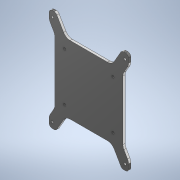
# Autodesk Inventor part: GPS - mount v2
Saved by Autodesk Inventor 2020.2 (Build 242310000, 310)
## iProperties
Created: 2020-08-26
Part Number: GPS - mount v2
Material: Generic
Document SubType Name: Modeling
Designer: Krishna Makhija
Density: 1 g/cm^3
Appearance: Default
Author: Krishna Makhija
Autodesk Inventor part; units mm, degrees
ref_plane "YZ Plane" through (0, 0, 0) normal (1, 0, 0) x (0, 1, 0)
ref_plane "XZ Plane" through (0, 0, 0) normal (0, 1, 0) x (-1, 0, 0)
ref_plane "XY Plane" through (0, 0, 0) normal (0, 0, 1) x (1, 0, 0)
sketch "Sketch3" plane through (0, 0, 0) normal (0, 0, 1) x (1, 0, 0)
  line L0 (52.5001, -67.5) -> (-52.5001, -67.5)
  line L1 (-52.5001, -67.5) -> (-52.5001, 67.5)
  line L2 (-52.5001, 67.5) -> (52.5001, 67.5)
  line L3 (52.5001, 67.5) -> (52.5001, -67.5)
  circle A0 centre (32, 32) radius 1.5
  circle A1 centre (-32, 32) radius 1.5
  circle A2 centre (-32, -32) radius 1.5
  circle A3 centre (32, -32) radius 1.5
  line L4 (30.5, 0) -> (-30.5, 0)
  line L5 (30.5, 45) -> (-30.5, 45)
  line L6 (30.5, 45) -> (43.4898, 67.5)
  line L7 (-30.5, 45) -> (-43.4888, 67.5)
  line L8 (30.5, -45) -> (-30.5, -45)
  line L9 (30.5, -45) -> (43.4898, -67.5)
  line L10 (-30.5, -45) -> (-43.4888, -67.5)
  line L11 (0, 42.0002) -> (0, -42)
  line L12 (45, 42.0002) -> (45, -42)
  line L13 (45, 42.0002) -> (52.5001, 54.9914)
  line L14 (45, -42) -> (52.5001, -54.9922)
  line L15 (-45, 42.0002) -> (-45, -42)
  line L16 (-45, 42.0002) -> (-52.5001, 54.9914)
  line L17 (-45, -42) -> (-52.5001, -54.9922)
  circle A4 centre (48, 60.0001) radius 1.428
  circle A5 centre (-48, 60.0001) radius 1.428
  circle A6 centre (48, -59.9999) radius 1.428
  circle A7 centre (-48, -59.9999) radius 1.428
  constraints: 36 end point, 8 centre point, 8 symmetric about line, 4 point on line, 3 horizontal, 2 parallel, 2 perpendicular
extrude "Extrusion2" add sketch "Sketch3" along normal blind 3 contours L0 L9 L8 L10 L1 L17 L15 L16 L2 L7 L5 L6 L3 L13 L12 L14 | L0 L10 L8 L9 | L14 L12 L13 L3 | L1 L16 L15 L17 | L6 L5 L7 L2 | A4 | A5 | A6 | A7
fillet "Fillet2" radius 4 4 edges at (-52.5001, 67.5, 1.5) (52.5001, 67.5, 1.5) (52.5001, -67.5, 1.5) (-52.5001, -67.5, 1.5)
extrude "Extrusion3" cut sketch "Sketch3" along normal blind 10 contours L0 L10 L8 L9 | L14 L12 L13 L3 | L1 L16 L15 L17 | L6 L5 L7 L2
fillet "Fillet3" radius 10 8 edges at (30.5, 45, 1.5) (-30.5, 45, 1.5) (30.5, -45, 1.5) (-30.5, -45, 1.5) (-52.5001, 54.9914, 1.5) (52.5001, -54.9922, 1.5) (-52.5001, -54.9922, 1.5) (52.5001, 54.9914, 1.5)
fillet "Fillet4" radius 10 4 edges at (45, 42.0002, 1.5) (45, -42, 1.5) (-45, -42, 1.5) (-45, 42.0002, 1.5)
fillet "Fillet5" radius 4 4 edges at (43.4898, 67.5, 1.5) (-43.4888, 67.5, 1.5) (43.4898, -67.5, 1.5) (-43.4888, -67.5, 1.5)
extrude "Extrusion4" cut sketch "Sketch3" along normal blind 10 contours A4 | A5 | A6 | A7
body "Solid2"
